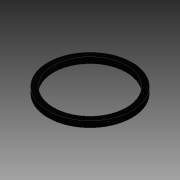
# Autodesk Inventor part: rubber
Saved by Autodesk Inventor 2014 SP1 (Build 180222100, 222)
## iProperties
Created: 2017-07-23
Part Number: rubber
Material: Типовые
Document SubType Name: Modeling
Designer: Stepan
Density: 1 g/cm^3
Appearance: Черный
Author: Stepan
Autodesk Inventor part; units mm, degrees
ref_plane "YZ Plane" through (0, 0, 0) normal (1, 0, 0) x (0, 1, 0)
ref_plane "XZ Plane" through (0, 0, 0) normal (0, 1, 0) x (-1, 0, 0)
sketch "Эскиз1" plane through (0, 0, 0) normal (0, 0, 1) x (1, 0, 0)
  circle A0 centre (-6.5, 0) radius 7.5 projected
  circle A1 centre (-6.5, 0) radius 6.5 projected
  point P0 (0, 0)
ref_plane "РабПлоскость1" through (-14, -7.5, 1.1) normal (0, 0, -1) x (0, 1, 0)
extrude "Выдавливание1" add sketch "Эскиз1" along normal up to surface (1.1 mm away)
fillet "Сопряжение1" radius 0.25 2 edges at (-14, 0, 1.1) (-14, 0, 0)
